Autodesk Inventor part; units mm, degrees
(part 2 of 2)
  spline S52 degree 2 poles (32.3634, 1.1115) (32.3453, 1.127) (32.3005, 1.138) (32.2753, 1.138) knots 0 0 0 1 2 2 2
  spline S53 degree 2 poles (32.2753, 1.138) (32.2539, 1.138) (32.2098, 1.127) (32.1903, 1.1192) knots 0 0 0 1 2 2 2
  spline S54 degree 2 poles (32.1903, 1.1192) (32.1903, 1.1141) (32.189, 1.0894) (32.189, 1.0706) knots 0 0 0 1 2 2 2
  spline S55 degree 2 poles (32.189, 1.0706) (32.189, 1.0013) (32.213, 0.9176) (32.2318, 0.8962) knots 0 0 0 1 2 2 2
  spline S56 degree 2 poles (32.2318, 0.8962) (32.2454, 0.8787) (32.2817, 0.8638) (32.3012, 0.8638) knots 0 0 0 1 2 2 2
  spline S57 degree 2 poles (32.3012, 0.8638) (32.3174, 0.8638) (32.355, 0.88) (32.368, 0.8962) knots 0 0 0 1 2 2 2
  line L247 (22.1174, -18.2657) -> (21.873, -18.2657)
  line L248 (21.873, -18.2657) -> (21.6506, -17.972)
  line L249 (21.6506, -17.972) -> (21.578, -17.972)
  line L250 (21.578, -17.972) -> (21.578, -18.2657)
  line L251 (21.578, -18.2657) -> (21.3784, -18.2657)
  line L252 (21.3784, -18.2657) -> (21.3784, -17.4657)
  line L253 (21.3784, -17.4657) -> (21.6999, -17.4657)
  spline S58 degree 2 poles (21.6999, -17.4657) (21.7667, -17.4657) (21.8652, -17.4826) (21.9074, -17.5085) knots 0 0 0 1 2 2 2
  spline S59 degree 2 poles (21.9074, -17.5085) (21.9502, -17.5357) (22.0007, -17.6206) (22.0007, -17.6855) knots 0 0 0 1 2 2 2
  spline S60 degree 2 poles (22.0007, -17.6855) (22.0007, -17.7769) (21.9177, -17.8916) (21.8484, -17.9253) knots 0 0 0 1 2 2 2
  line L254 (21.8484, -17.9253) -> (22.1174, -18.2657)
  spline S61 degree 2 poles (21.7946, -17.7108) (21.7946, -17.6803) (21.7712, -17.6368) (21.7446, -17.6252) knots 0 0 0 1 2 2 2
  spline S62 degree 2 poles (21.7446, -17.6252) (21.7258, -17.6174) (21.6798, -17.6129) (21.6455, -17.6129) knots 0 0 0 1 2 2 2
  line L255 (21.6455, -17.6129) -> (21.578, -17.6129)
  line L256 (21.578, -17.6129) -> (21.578, -17.8281)
  line L257 (21.578, -17.8281) -> (21.6357, -17.8281)
  spline S63 degree 2 poles (21.6357, -17.8281) (21.6772, -17.8281) (21.7362, -17.8177) (21.7563, -17.8015) knots 0 0 0 1 2 2 2
  spline S64 degree 2 poles (21.7563, -17.8015) (21.7758, -17.786) (21.7946, -17.7445) (21.7946, -17.7108) knots 0 0 0 1 2 2 2
  line L258 (22.7275, -18.2657) -> (22.1991, -18.2657)
  line L259 (22.1991, -18.2657) -> (22.1991, -18.1263)
  line L260 (22.1991, -18.1263) -> (22.3677, -18.1263)
  line L261 (22.3677, -18.1263) -> (22.3677, -17.703)
  line L262 (22.3677, -17.703) -> (22.1991, -17.703)
  line L263 (22.1991, -17.703) -> (22.1991, -17.5727)
  spline S65 degree 2 poles (22.1991, -17.5727) (22.2361, -17.5727) (22.3093, -17.5629) (22.3314, -17.5526) knots 0 0 0 1 2 2 2
  spline S66 degree 2 poles (22.3314, -17.5526) (22.3566, -17.5396) (22.3852, -17.4962) (22.3878, -17.4638) knots 0 0 0 1 2 2 2
  line L264 (22.3878, -17.4638) -> (22.5628, -17.4638)
  line L265 (22.5628, -17.4638) -> (22.5628, -18.1263)
  line L266 (22.5628, -18.1263) -> (22.7275, -18.1263)
  line L267 (22.7275, -18.1263) -> (22.7275, -18.2657)
  spline S67 degree 2 poles (22.1278, -9.1391) (22.1278, -9.1909) (22.0922, -9.283) (22.0565, -9.3154) knots 0 0 0 1 2 2 2
  spline S68 degree 2 poles (22.0565, -9.3154) (22.0163, -9.3517) (21.9068, -9.3861) (21.8354, -9.3861) knots 0 0 0 1 2 2 2
  spline S69 degree 2 poles (21.8354, -9.3861) (21.7823, -9.3861) (21.6889, -9.3783) (21.6533, -9.3705) knots 0 0 0 1 2 2 2
  line L268 (21.6533, -9.3705) -> (21.6533, -9.2084)
  line L269 (21.6533, -9.2084) -> (21.6714, -9.2084)
  spline S70 degree 2 poles (21.6714, -9.2084) (21.6954, -9.2182) (21.7479, -9.235) (21.7894, -9.235) knots 0 0 0 1 2 2 2
  spline S71 degree 2 poles (21.7894, -9.235) (21.8426, -9.235) (21.9003, -9.2052) (21.9119, -9.178) knots 0 0 0 1 2 2 2
  spline S72 degree 2 poles (21.9119, -9.178) (21.9243, -9.1514) (21.9268, -9.0827) (21.9268, -9.0399) knots 0 0 0 1 2 2 2
  line L270 (21.9268, -9.0399) -> (21.9268, -8.719)
  line L271 (21.9268, -8.719) -> (21.744, -8.719)
  line L272 (21.744, -8.719) -> (21.744, -8.5738)
  line L273 (21.744, -8.5738) -> (22.1278, -8.5738)
  line L274 (22.1278, -8.5738) -> (22.1278, -9.1391)
  line L275 (22.8695, -9.3738) -> (22.2815, -9.3738)
  line L276 (22.2815, -9.3738) -> (22.2815, -9.2435)
  spline S73 degree 2 poles (22.2815, -9.2435) (22.356, -9.1838) (22.4753, -9.0788) (22.52, -9.0315) knots 0 0 0 1 2 2 2
  spline S74 degree 2 poles (22.52, -9.0315) (22.579, -8.9699) (22.6315, -8.8759) (22.6315, -8.8266) knots 0 0 0 1 2 2 2
  spline S75 degree 2 poles (22.6315, -8.8266) (22.6315, -8.7708) (22.5648, -8.7112) (22.5051, -8.7112) knots 0 0 0 1 2 2 2
  spline S76 degree 2 poles (22.5051, -8.7112) (22.4747, -8.7112) (22.4202, -8.7261) (22.3923, -8.7378) knots 0 0 0 1 2 2 2
  spline S77 degree 2 poles (22.3923, -8.7378) (22.3651, -8.7501) (22.3262, -8.776) (22.3165, -8.7825) knots 0 0 0 1 2 2 2
  line L277 (22.3165, -8.7825) -> (22.3009, -8.7825)
  line L278 (22.3009, -8.7825) -> (22.3009, -8.6081)
  spline S78 degree 2 poles (22.3009, -8.6081) (22.3346, -8.5919) (22.4786, -8.5582) (22.5453, -8.5582) knots 0 0 0 1 2 2 2
  spline S79 degree 2 poles (22.5453, -8.5582) (22.688, -8.5582) (22.8345, -8.6853) (22.8345, -8.8) knots 0 0 0 1 2 2 2
  spline S80 degree 2 poles (22.8345, -8.8) (22.8345, -8.8707) (22.7677, -9.0068) (22.6905, -9.0846) knots 0 0 0 1 2 2 2
  spline S81 degree 2 poles (22.6905, -9.0846) (22.6419, -9.1326) (22.5505, -9.2072) (22.5304, -9.2227) knots 0 0 0 1 2 2 2
  line L279 (22.5304, -9.2227) -> (22.8695, -9.2227)
  line L280 (22.8695, -9.2227) -> (22.8695, -9.3738)
  spline S82 degree 2 poles (20.6809, -6.6196) (20.6809, -6.6715) (20.6452, -6.7636) (20.6096, -6.796) knots 0 0 0 1 2 2 2
  spline S83 degree 2 poles (20.6096, -6.796) (20.5694, -6.8323) (20.4598, -6.8667) (20.3885, -6.8667) knots 0 0 0 1 2 2 2
  spline S84 degree 2 poles (20.3885, -6.8667) (20.3353, -6.8667) (20.242, -6.8589) (20.2063, -6.8511) knots 0 0 0 1 2 2 2
  line L281 (20.2063, -6.8511) -> (20.2063, -6.689)
  line L282 (20.2063, -6.689) -> (20.2245, -6.689)
  spline S85 degree 2 poles (20.2245, -6.689) (20.2485, -6.6987) (20.301, -6.7156) (20.3425, -6.7156) knots 0 0 0 1 2 2 2
  spline S86 degree 2 poles (20.3425, -6.7156) (20.3956, -6.7156) (20.4533, -6.6858) (20.465, -6.6585) knots 0 0 0 1 2 2 2
  spline S87 degree 2 poles (20.465, -6.6585) (20.4773, -6.632) (20.4799, -6.5632) (20.4799, -6.5205) knots 0 0 0 1 2 2 2
  line L283 (20.4799, -6.5205) -> (20.4799, -6.1996)
  line L284 (20.4799, -6.1996) -> (20.2971, -6.1996)
  line L285 (20.2971, -6.1996) -> (20.2971, -6.0543)
  line L286 (20.2971, -6.0543) -> (20.6809, -6.0543)
  line L287 (20.6809, -6.0543) -> (20.6809, -6.6196)
  line L288 (21.3869, -6.8543) -> (20.8585, -6.8543)
  line L289 (20.8585, -6.8543) -> (20.8585, -6.7149)
  line L290 (20.8585, -6.7149) -> (21.0271, -6.7149)
  line L291 (21.0271, -6.7149) -> (21.0271, -6.2916)
  line L292 (21.0271, -6.2916) -> (20.8585, -6.2916)
  line L293 (20.8585, -6.2916) -> (20.8585, -6.1613)
  spline S88 degree 2 poles (20.8585, -6.1613) (20.8955, -6.1613) (20.9687, -6.1516) (20.9908, -6.1412) knots 0 0 0 1 2 2 2
  spline S89 degree 2 poles (20.9908, -6.1412) (21.016, -6.1282) (21.0446, -6.0848) (21.0472, -6.0524) knots 0 0 0 1 2 2 2
  line L294 (21.0472, -6.0524) -> (21.2222, -6.0524)
  line L295 (21.2222, -6.0524) -> (21.2222, -6.7149)
  line L296 (21.2222, -6.7149) -> (21.3869, -6.7149)
  line L297 (21.3869, -6.7149) -> (21.3869, -6.8543)
  line L298 (22.4777, 11.6258) -> (22.2333, 11.6258)
  line L299 (22.2333, 11.6258) -> (22.0109, 11.9195)
  line L300 (22.0109, 11.9195) -> (21.9383, 11.9195)
  line L301 (21.9383, 11.9195) -> (21.9383, 11.6258)
  line L302 (21.9383, 11.6258) -> (21.7386, 11.6258)
  line L303 (21.7386, 11.6258) -> (21.7386, 12.4258)
  line L304 (21.7386, 12.4258) -> (22.0602, 12.4258)
  spline S90 degree 2 poles (22.0602, 12.4258) (22.127, 12.4258) (22.2255, 12.4089) (22.2676, 12.383) knots 0 0 0 1 2 2 2
  spline S91 degree 2 poles (22.2676, 12.383) (22.3104, 12.3558) (22.361, 12.2709) (22.361, 12.206) knots 0 0 0 1 2 2 2
  spline S92 degree 2 poles (22.361, 12.206) (22.361, 12.1146) (22.278, 11.9999) (22.2086, 11.9662) knots 0 0 0 1 2 2 2
  line L305 (22.2086, 11.9662) -> (22.4777, 11.6258)
  spline S93 degree 2 poles (22.1548, 12.1807) (22.1548, 12.2112) (22.1315, 12.2547) (22.1049, 12.2663) knots 0 0 0 1 2 2 2
  spline S94 degree 2 poles (22.1049, 12.2663) (22.0861, 12.2741) (22.0401, 12.2786) (22.0057, 12.2786) knots 0 0 0 1 2 2 2
  line L306 (22.0057, 12.2786) -> (21.9383, 12.2786)
  line L307 (21.9383, 12.2786) -> (21.9383, 12.0634)
  line L308 (21.9383, 12.0634) -> (21.996, 12.0634)
  spline S95 degree 2 poles (21.996, 12.0634) (22.0375, 12.0634) (22.0965, 12.0738) (22.1166, 12.09) knots 0 0 0 1 2 2 2
  spline S96 degree 2 poles (22.1166, 12.09) (22.136, 12.1055) (22.1548, 12.147) (22.1548, 12.1807) knots 0 0 0 1 2 2 2
  line L309 (23.1234, 11.6258) -> (22.5354, 11.6258)
  line L310 (22.5354, 11.6258) -> (22.5354, 11.7561)
  spline S97 degree 2 poles (22.5354, 11.7561) (22.6099, 11.8158) (22.7292, 11.9208) (22.774, 11.9681) knots 0 0 0 1 2 2 2
  spline S98 degree 2 poles (22.774, 11.9681) (22.833, 12.0297) (22.8855, 12.1237) (22.8855, 12.173) knots 0 0 0 1 2 2 2
  spline S99 degree 2 poles (22.8855, 12.173) (22.8855, 12.2287) (22.8187, 12.2884) (22.759, 12.2884) knots 0 0 0 1 2 2 2
  spline S100 degree 2 poles (22.759, 12.2884) (22.7286, 12.2884) (22.6741, 12.2735) (22.6462, 12.2618) knots 0 0 0 1 2 2 2
  spline S101 degree 2 poles (22.6462, 12.2618) (22.619, 12.2495) (22.5801, 12.2235) (22.5704, 12.217) knots 0 0 0 1 2 2 2
  line L311 (22.5704, 12.217) -> (22.5548, 12.217)
  line L312 (22.5548, 12.217) -> (22.5548, 12.3914)
  spline S102 degree 2 poles (22.5548, 12.3914) (22.5885, 12.4076) (22.7325, 12.4414) (22.7992, 12.4414) knots 0 0 0 1 2 2 2
  spline S103 degree 2 poles (22.7992, 12.4414) (22.9419, 12.4414) (23.0884, 12.3143) (23.0884, 12.1995) knots 0 0 0 1 2 2 2
  spline S104 degree 2 poles (23.0884, 12.1995) (23.0884, 12.1289) (23.0216, 11.9927) (22.9445, 11.9149) knots 0 0 0 1 2 2 2
  spline S105 degree 2 poles (22.9445, 11.9149) (22.8958, 11.867) (22.8044, 11.7924) (22.7843, 11.7769) knots 0 0 0 1 2 2 2
  line L313 (22.7843, 11.7769) -> (23.1234, 11.7769)
  line L314 (23.1234, 11.7769) -> (23.1234, 11.6258)
  line L315 (40.1797, -0.8005) -> (40.45, -0.0005)
  line L316 (40.45, -0.0005) -> (40.6692, -0.0005)
  line L317 (40.6692, -0.0005) -> (40.9395, -0.8005)
  line L318 (40.9395, -0.8005) -> (40.7327, -0.8005)
  line L319 (40.7327, -0.8005) -> (40.6828, -0.6371)
  line L320 (40.6828, -0.6371) -> (40.4312, -0.6371)
  line L321 (40.4312, -0.6371) -> (40.3807, -0.8005)
  line L322 (40.3807, -0.8005) -> (40.1797, -0.8005)
  line L323 (40.6387, -0.4919) -> (40.557, -0.2274)
  line L324 (40.557, -0.2274) -> (40.4747, -0.4919)
  line L325 (40.4747, -0.4919) -> (40.6387, -0.4919)
  line L326 (41.0192, -0.8005) -> (41.0192, -0.0005)
  line L327 (41.0192, -0.0005) -> (41.5599, -0.0005)
  line L328 (41.5599, -0.0005) -> (41.5599, -0.1528)
  line L329 (41.5599, -0.1528) -> (41.2189, -0.1528)
  line L330 (41.2189, -0.1528) -> (41.2189, -0.2935)
  line L331 (41.2189, -0.2935) -> (41.5333, -0.2935)
  line L332 (41.5333, -0.2935) -> (41.5333, -0.4459)
  line L333 (41.5333, -0.4459) -> (41.2189, -0.4459)
  line L334 (41.2189, -0.4459) -> (41.2189, -0.6481)
  line L335 (41.2189, -0.6481) -> (41.5599, -0.6481)
  line L336 (41.5599, -0.6481) -> (41.5599, -0.8005)
  line L337 (41.5599, -0.8005) -> (41.0192, -0.8005)
  line L338 (42.2821, -0.8005) -> (41.6941, -0.8005)
  line L339 (41.6941, -0.8005) -> (41.6941, -0.6702)
  spline S106 degree 2 poles (41.6941, -0.6702) (41.7687, -0.6105) (41.888, -0.5055) (41.9327, -0.4582) knots 0 0 0 1 2 2 2
  spline S107 degree 2 poles (41.9327, -0.4582) (41.9917, -0.3966) (42.0442, -0.3026) (42.0442, -0.2533) knots 0 0 0 1 2 2 2
  spline S108 degree 2 poles (42.0442, -0.2533) (42.0442, -0.1976) (41.9774, -0.1379) (41.9178, -0.1379) knots 0 0 0 1 2 2 2
  spline S109 degree 2 poles (41.9178, -0.1379) (41.8873, -0.1379) (41.8329, -0.1528) (41.805, -0.1645) knots 0 0 0 1 2 2 2
  spline S110 degree 2 poles (41.805, -0.1645) (41.7778, -0.1768) (41.7389, -0.2027) (41.7291, -0.2092) knots 0 0 0 1 2 2 2
  line L340 (41.7291, -0.2092) -> (41.7136, -0.2092)
  line L341 (41.7136, -0.2092) -> (41.7136, -0.0348)
  spline S111 degree 2 poles (41.7136, -0.0348) (41.7473, -0.0186) (41.8912, 0.0151) (41.958, 0.0151) knots 0 0 0 1 2 2 2
  spline S112 degree 2 poles (41.958, 0.0151) (42.1006, 0.0151) (42.2471, -0.112) (42.2471, -0.2267) knots 0 0 0 1 2 2 2
  spline S113 degree 2 poles (42.2471, -0.2267) (42.2471, -0.2974) (42.1803, -0.4335) (42.1032, -0.5113) knots 0 0 0 1 2 2 2
  spline S114 degree 2 poles (42.1032, -0.5113) (42.0546, -0.5593) (41.9632, -0.6339) (41.9431, -0.6494) knots 0 0 0 1 2 2 2
  line L342 (41.9431, -0.6494) -> (42.2821, -0.6494)
  line L343 (42.2821, -0.6494) -> (42.2821, -0.8005)
  line L344 (44.752, -28.4247) -> (44.551, -28.4247)
  line L345 (44.551, -28.4247) -> (44.551, -28.07)
  line L346 (44.551, -28.07) -> (44.2781, -28.07)
  line L347 (44.2781, -28.07) -> (44.2781, -28.4247)
  line L348 (44.2781, -28.4247) -> (44.0771, -28.4247)
  line L349 (44.0771, -28.4247) -> (44.0771, -27.6247)
  line L350 (44.0771, -27.6247) -> (44.2781, -27.6247)
  line L351 (44.2781, -27.6247) -> (44.2781, -27.9177)
  line L352 (44.2781, -27.9177) -> (44.551, -27.9177)
  line L353 (44.551, -27.9177) -> (44.551, -27.6247)
  line L354 (44.551, -27.6247) -> (44.752, -27.6247)
  line L355 (44.752, -27.6247) -> (44.752, -28.4247)
  line L356 (45.4865, -27.7835) -> (45.1449, -28.4247)
  line L357 (45.1449, -28.4247) -> (44.9219, -28.4247)
  line L358 (44.9219, -28.4247) -> (45.2791, -27.7757)
  line L359 (45.2791, -27.7757) -> (44.8979, -27.7757)
  line L360 (44.8979, -27.7757) -> (44.8979, -27.6247)
  line L361 (44.8979, -27.6247) -> (45.4865, -27.6247)
  line L362 (45.4865, -27.6247) -> (45.4865, -27.7835)
  line L363 (44.8169, 27.8958) -> (44.6159, 27.8958)
  line L364 (44.6159, 27.8958) -> (44.6159, 28.2505)
  line L365 (44.6159, 28.2505) -> (44.3429, 28.2505)
  line L366 (44.3429, 28.2505) -> (44.3429, 27.8958)
  line L367 (44.3429, 27.8958) -> (44.142, 27.8958)
  line L368 (44.142, 27.8958) -> (44.142, 28.6958)
  line L369 (44.142, 28.6958) -> (44.3429, 28.6958)
  line L370 (44.3429, 28.6958) -> (44.3429, 28.4028)
  line L371 (44.3429, 28.4028) -> (44.6159, 28.4028)
  line L372 (44.6159, 28.4028) -> (44.6159, 28.6958)
  line L373 (44.6159, 28.6958) -> (44.8169, 28.6958)
  line L374 (44.8169, 28.6958) -> (44.8169, 27.8958)
  spline S115 degree 2 poles (45.5669, 28.1182) (45.5669, 28.067) (45.5241, 27.9782) (45.4833, 27.9458) knots 0 0 0 1 2 2 2
  spline S116 degree 2 poles (45.4833, 27.9458) (45.4425, 27.9133) (45.3251, 27.877) (45.2493, 27.877) knots 0 0 0 1 2 2 2
  spline S117 degree 2 poles (45.2493, 27.877) (45.1682, 27.877) (45.047, 27.914) (45.0081, 27.9458) knots 0 0 0 1 2 2 2
  spline S118 degree 2 poles (45.0081, 27.9458) (44.9699, 27.9775) (44.9335, 28.0637) (44.9335, 28.1117) knots 0 0 0 1 2 2 2
  spline S119 degree 2 poles (44.9335, 28.1117) (44.9335, 28.1804) (45.0094, 28.2719) (45.0814, 28.3023) knots 0 0 0 1 2 2 2
  line L375 (45.0814, 28.3023) -> (45.0814, 28.3056)
  spline S120 degree 2 poles (45.0814, 28.3056) (45.0107, 28.3399) (44.9549, 28.4378) (44.9549, 28.4981) knots 0 0 0 1 2 2 2
  spline S121 degree 2 poles (44.9549, 28.4981) (44.9549, 28.5422) (44.9938, 28.6193) (45.0321, 28.6498) knots 0 0 0 1 2 2 2
  spline S122 degree 2 poles (45.0321, 28.6498) (45.069, 28.679) (45.1812, 28.714) (45.2512, 28.714) knots 0 0 0 1 2 2 2
  spline S123 degree 2 poles (45.2512, 28.714) (45.3251, 28.714) (45.4353, 28.6822) (45.471, 28.6563) knots 0 0 0 1 2 2 2
  spline S124 degree 2 poles (45.471, 28.6563) (45.5073, 28.6304) (45.5462, 28.5552) (45.5462, 28.5117) knots 0 0 0 1 2 2 2
  spline S125 degree 2 poles (45.5462, 28.5117) (45.5462, 28.4547) (45.4801, 28.3633) (45.412, 28.3315) knots 0 0 0 1 2 2 2
  line L376 (45.412, 28.3315) -> (45.412, 28.3289)
  spline S126 degree 2 poles (45.412, 28.3289) (45.4917, 28.2965) (45.5669, 28.1915) (45.5669, 28.1182) knots 0 0 0 1 2 2 2
  spline S127 degree 2 poles (45.3686, 28.1098) (45.3686, 28.1493) (45.3348, 28.1908) (45.2804, 28.2174) knots 0 0 0 1 2 2 2
  spline S128 degree 2 poles (45.2804, 28.2174) (45.2648, 28.2245) (45.2058, 28.2472) (45.1831, 28.2569) knots 0 0 0 1 2 2 2
  spline S129 degree 2 poles (45.1831, 28.2569) (45.1624, 28.2362) (45.1293, 28.174) (45.1293, 28.137) knots 0 0 0 1 2 2 2
  spline S130 degree 2 poles (45.1293, 28.137) (45.1293, 28.0813) (45.2006, 28.0145) (45.2583, 28.0145) knots 0 0 0 1 2 2 2
  spline S131 degree 2 poles (45.2583, 28.0145) (45.2746, 28.0145) (45.3147, 28.0249) (45.3303, 28.0352) knots 0 0 0 1 2 2 2
  spline S132 degree 2 poles (45.3303, 28.0352) (45.3478, 28.0475) (45.3686, 28.0813) (45.3686, 28.1098) knots 0 0 0 1 2 2 2
  spline S133 degree 2 poles (45.3511, 28.4884) (45.3511, 28.5292) (45.2972, 28.5778) (45.2512, 28.5778) knots 0 0 0 1 2 2 2
  spline S134 degree 2 poles (45.2512, 28.5778) (45.2071, 28.5778) (45.1533, 28.5338) (45.1533, 28.5013) knots 0 0 0 1 2 2 2
  spline S135 degree 2 poles (45.1533, 28.5013) (45.1533, 28.4696) (45.1857, 28.43) (45.2201, 28.4138) knots 0 0 0 1 2 2 2
  spline S136 degree 2 poles (45.2201, 28.4138) (45.235, 28.406) (45.2765, 28.3898) (45.3109, 28.3769) knots 0 0 0 1 2 2 2
  spline S137 degree 2 poles (45.3109, 28.3769) (45.3316, 28.4041) (45.3511, 28.4553) (45.3511, 28.4884) knots 0 0 0 1 2 2 2
  line L377 (-8.7757, -9.36) -> (-8.5053, -8.56)
  line L378 (-8.5053, -8.56) -> (-8.2862, -8.56)
  line L379 (-8.2862, -8.56) -> (-8.0159, -9.36)
  line L380 (-8.0159, -9.36) -> (-8.2227, -9.36)
  line L381 (-8.2227, -9.36) -> (-8.2726, -9.1966)
  line L382 (-8.2726, -9.1966) -> (-8.5241, -9.1966)
  line L383 (-8.5241, -9.1966) -> (-8.5747, -9.36)
  line L384 (-8.5747, -9.36) -> (-8.7757, -9.36)
  line L385 (-8.3167, -9.0514) -> (-8.3983, -8.7869)
  line L386 (-8.3983, -8.7869) -> (-8.4807, -9.0514)
  line L387 (-8.4807, -9.0514) -> (-8.3167, -9.0514)
  line L388 (-7.9361, -9.36) -> (-7.9361, -8.56)
  line L389 (-7.9361, -8.56) -> (-7.3954, -8.56)
  line L390 (-7.3954, -8.56) -> (-7.3954, -8.7123)
  line L391 (-7.3954, -8.7123) -> (-7.7364, -8.7123)
  line L392 (-7.7364, -8.7123) -> (-7.7364, -8.853)
  line L393 (-7.7364, -8.853) -> (-7.422, -8.853)
  line L394 (-7.422, -8.853) -> (-7.422, -9.0053)
  line L395 (-7.422, -9.0053) -> (-7.7364, -9.0053)
  line L396 (-7.7364, -9.0053) -> (-7.7364, -9.2076)
  line L397 (-7.7364, -9.2076) -> (-7.3954, -9.2076)
  line L398 (-7.3954, -9.2076) -> (-7.3954, -9.36)
  line L399 (-7.3954, -9.36) -> (-7.9361, -9.36)
  line L400 (-6.7089, -9.36) -> (-7.2372, -9.36)
  line L401 (-7.2372, -9.36) -> (-7.2372, -9.2206)
  line L402 (-7.2372, -9.2206) -> (-7.0687, -9.2206)
  line L403 (-7.0687, -9.2206) -> (-7.0687, -8.7972)
  line L404 (-7.0687, -8.7972) -> (-7.2372, -8.7972)
  line L405 (-7.2372, -8.7972) -> (-7.2372, -8.6669)
  spline S138 degree 2 poles (-7.2372, -8.6669) (-7.2003, -8.6669) (-7.127, -8.6572) (-7.105, -8.6468) knots 0 0 0 1 2 2 2
  spline S139 degree 2 poles (-7.105, -8.6468) (-7.0797, -8.6339) (-7.0512, -8.5904) (-7.0486, -8.558) knots 0 0 0 1 2 2 2
  line L406 (-7.0486, -8.558) -> (-6.8735, -8.558)
  line L407 (-6.8735, -8.558) -> (-6.8735, -9.2206)
  line L408 (-6.8735, -9.2206) -> (-6.7089, -9.2206)
  line L409 (-6.7089, -9.2206) -> (-6.7089, -9.36)
  line L410 (-23.6301, 21.6881) -> (-23.831, 21.6881)
  line L411 (-23.831, 21.6881) -> (-23.831, 22.0427)
  line L412 (-23.831, 22.0427) -> (-24.104, 22.0427)
  line L413 (-24.104, 22.0427) -> (-24.104, 21.6881)
  line L414 (-24.104, 21.6881) -> (-24.3049, 21.6881)
  line L415 (-24.3049, 21.6881) -> (-24.3049, 22.4881)
  line L416 (-24.3049, 22.4881) -> (-24.104, 22.4881)
  line L417 (-24.104, 22.4881) -> (-24.104, 22.195)
  line L418 (-24.104, 22.195) -> (-23.831, 22.195)
  line L419 (-23.831, 22.195) -> (-23.831, 22.4881)
  line L420 (-23.831, 22.4881) -> (-23.6301, 22.4881)
  line L421 (-23.6301, 22.4881) -> (-23.6301, 21.6881)
  line L422 (-22.8683, 21.8748) -> (-22.9766, 21.8748)
  line L423 (-22.9766, 21.8748) -> (-22.9766, 21.6861)
  line L424 (-22.9766, 21.6861) -> (-23.1704, 21.6861)
  line L425 (-23.1704, 21.6861) -> (-23.1704, 21.8748)
  line L426 (-23.1704, 21.8748) -> (-23.5231, 21.8748)
  line L427 (-23.5231, 21.8748) -> (-23.5231, 22.0239)
  line L428 (-23.5231, 22.0239) -> (-23.1769, 22.4881)
  line L429 (-23.1769, 22.4881) -> (-22.9766, 22.4881)
  line L430 (-22.9766, 22.4881) -> (-22.9766, 22.0187)
  line L431 (-22.9766, 22.0187) -> (-22.8683, 22.0187)
  line L432 (-22.8683, 22.0187) -> (-22.8683, 21.8748)
  line L433 (-23.1704, 22.0187) -> (-23.1704, 22.291)
  line L434 (-23.1704, 22.291) -> (-23.3733, 22.0187)
  line L435 (-23.3733, 22.0187) -> (-23.1704, 22.0187)
  line L436 (-23.5442, -22.2943) -> (-23.7451, -22.2943)
  line L437 (-23.7451, -22.2943) -> (-23.7451, -21.9397)
  line L438 (-23.7451, -21.9397) -> (-24.0181, -21.9397)
  line L439 (-24.0181, -21.9397) -> (-24.0181, -22.2943)
  line L440 (-24.0181, -22.2943) -> (-24.219, -22.2943)
  line L441 (-24.219, -22.2943) -> (-24.219, -21.4943)
  line L442 (-24.219, -21.4943) -> (-24.0181, -21.4943)
  line L443 (-24.0181, -21.4943) -> (-24.0181, -21.7873)
  line L444 (-24.0181, -21.7873) -> (-23.7451, -21.7873)
  line L445 (-23.7451, -21.7873) -> (-23.7451, -21.4943)
  line L446 (-23.7451, -21.4943) -> (-23.5442, -21.4943)
  line L447 (-23.5442, -21.4943) -> (-23.5442, -22.2943)
  spline S140 degree 2 poles (-22.8122, -22.0518) (-22.8122, -22.1108) (-22.8557, -22.2074) (-22.8978, -22.2411) knots 0 0 0 1 2 2 2
  spline S141 degree 2 poles (-22.8978, -22.2411) (-22.94, -22.2749) (-23.0547, -22.3112) (-23.137, -22.3112) knots 0 0 0 1 2 2 2
  spline S142 degree 2 poles (-23.137, -22.3112) (-23.2304, -22.3112) (-23.3639, -22.28) (-23.4061, -22.2606) knots 0 0 0 1 2 2 2
  line L448 (-23.4061, -22.2606) -> (-23.4061, -22.0868)
  line L449 (-23.4061, -22.0868) -> (-23.3866, -22.0868)
  spline S143 degree 2 poles (-23.3866, -22.0868) (-23.3425, -22.1147) (-23.2239, -22.1562) (-23.1746, -22.1562) knots 0 0 0 1 2 2 2
  spline S144 degree 2 poles (-23.1746, -22.1562) (-23.1455, -22.1562) (-23.0774, -22.1458) (-23.0541, -22.129) knots 0 0 0 1 2 2 2
  spline S145 degree 2 poles (-23.0541, -22.129) (-23.0359, -22.1154) (-23.0139, -22.0758) (-23.0139, -22.0402) knots 0 0 0 1 2 2 2
  spline S146 degree 2 poles (-23.0139, -22.0402) (-23.0139, -22.0045) (-23.045, -21.9663) (-23.0709, -21.9572) knots 0 0 0 1 2 2 2
  spline S147 degree 2 poles (-23.0709, -21.9572) (-23.0968, -21.9481) (-23.1688, -21.9462) (-23.1967, -21.9462) knots 0 0 0 1 2 2 2
  line L450 (-23.1967, -21.9462) -> (-23.231, -21.9462)
  line L451 (-23.231, -21.9462) -> (-23.231, -21.8055)
  line L452 (-23.231, -21.8055) -> (-23.1993, -21.8055)
  spline S148 degree 2 poles (-23.1993, -21.8055) (-23.163, -21.8055) (-23.1014, -21.799) (-23.08, -21.7893) knots 0 0 0 1 2 2 2
  spline S149 degree 2 poles (-23.08, -21.7893) (-23.0586, -21.7789) (-23.0346, -21.7426) (-23.0346, -21.7115) knots 0 0 0 1 2 2 2
  spline S150 degree 2 poles (-23.0346, -21.7115) (-23.0346, -21.6868) (-23.0573, -21.6564) (-23.0735, -21.6479) knots 0 0 0 1 2 2 2
  spline S151 degree 2 poles (-23.0735, -21.6479) (-23.093, -21.6382) (-23.1448, -21.6317) (-23.163, -21.6317) knots 0 0 0 1 2 2 2
  spline S152 degree 2 poles (-23.163, -21.6317) (-23.1921, -21.6317) (-23.2537, -21.6454) (-23.2823, -21.6564) knots 0 0 0 1 2 2 2
  spline S153 degree 2 poles (-23.2823, -21.6564) (-23.3049, -21.6648) (-23.3542, -21.692) (-23.3659, -21.6992) knots 0 0 0 1 2 2 2
  line L453 (-23.3659, -21.6992) -> (-23.3827, -21.6992)
  line L454 (-23.3827, -21.6992) -> (-23.3827, -21.528)
  spline S154 degree 2 poles (-23.3827, -21.528) (-23.3413, -21.5105) (-23.2012, -21.4774) (-23.128, -21.4774) knots 0 0 0 1 2 2 2
  spline S155 degree 2 poles (-23.128, -21.4774) (-23.0566, -21.4774) (-22.9516, -21.5021) (-22.9147, -21.5261) knots 0 0 0 1 2 2 2
  spline S156 degree 2 poles (-22.9147, -21.5261) (-22.8738, -21.5514) (-22.833, -21.6291) (-22.833, -21.6778) knots 0 0 0 1 2 2 2
  spline S157 degree 2 poles (-22.833, -21.6778) (-22.833, -21.7465) (-22.9121, -21.8489) (-22.9769, -21.8638) knots 0 0 0 1 2 2 2
  line L455 (-22.9769, -21.8638) -> (-22.9769, -21.8716)
  spline S158 degree 2 poles (-22.9769, -21.8716) (-22.9484, -21.8755) (-22.8939, -21.8962) (-22.868, -21.9196) knots 0 0 0 1 2 2 2
  spline S159 degree 2 poles (-22.868, -21.9196) (-22.844, -21.9403) (-22.8122, -22.0065) (-22.8122, -22.0518) knots 0 0 0 1 2 2 2
  line L456 (-45.2027, -28.4422) -> (-45.4037, -28.4422)
  line L457 (-45.4037, -28.4422) -> (-45.4037, -28.0876)
  line L458 (-45.4037, -28.0876) -> (-45.6766, -28.0876)
  line L459 (-45.6766, -28.0876) -> (-45.6766, -28.4422)
  line L460 (-45.6766, -28.4422) -> (-45.8776, -28.4422)
  line L461 (-45.8776, -28.4422) -> (-45.8776, -27.6422)
  line L462 (-45.8776, -27.6422) -> (-45.6766, -27.6422)
  line L463 (-45.6766, -27.6422) -> (-45.6766, -27.9353)
  line L464 (-45.6766, -27.9353) -> (-45.4037, -27.9353)
  line L465 (-45.4037, -27.9353) -> (-45.4037, -27.6422)
  line L466 (-45.4037, -27.6422) -> (-45.2027, -27.6422)
  line L467 (-45.2027, -27.6422) -> (-45.2027, -28.4422)
  line L468 (-44.4863, -28.4422) -> (-45.0147, -28.4422)
  line L469 (-45.0147, -28.4422) -> (-45.0147, -28.3028)
  line L470 (-45.0147, -28.3028) -> (-44.8461, -28.3028)
  line L471 (-44.8461, -28.3028) -> (-44.8461, -27.8795)
  line L472 (-44.8461, -27.8795) -> (-45.0147, -27.8795)
  line L473 (-45.0147, -27.8795) -> (-45.0147, -27.7492)
  spline S160 degree 2 poles (-45.0147, -27.7492) (-44.9777, -27.7492) (-44.9045, -27.7395) (-44.8824, -27.7291) knots 0 0 0 1 2 2 2
  spline S161 degree 2 poles (-44.8824, -27.7291) (-44.8571, -27.7161) (-44.8286, -27.6727) (-44.826, -27.6403) knots 0 0 0 1 2 2 2
  line L474 (-44.826, -27.6403) -> (-44.651, -27.6403)
  line L475 (-44.651, -27.6403) -> (-44.651, -28.3028)
  line L476 (-44.651, -28.3028) -> (-44.4863, -28.3028)
  line L477 (-44.4863, -28.3028) -> (-44.4863, -28.4422)
  line L478 (-45.5229, 27.6078) -> (-45.7239, 27.6078)
  line L479 (-45.7239, 27.6078) -> (-45.7239, 27.9624)
  line L480 (-45.7239, 27.9624) -> (-45.9968, 27.9624)
  line L481 (-45.9968, 27.9624) -> (-45.9968, 27.6078)
  line L482 (-45.9968, 27.6078) -> (-46.1978, 27.6078)
  line L483 (-46.1978, 27.6078) -> (-46.1978, 28.4078)
  line L484 (-46.1978, 28.4078) -> (-45.9968, 28.4078)
  line L485 (-45.9968, 28.4078) -> (-45.9968, 28.1147)
  line L486 (-45.9968, 28.1147) -> (-45.7239, 28.1147)
  line L487 (-45.7239, 28.1147) -> (-45.7239, 28.4078)
  line L488 (-45.7239, 28.4078) -> (-45.5229, 28.4078)
  line L489 (-45.5229, 28.4078) -> (-45.5229, 27.6078)
  line L490 (-44.7709, 27.6078) -> (-45.3589, 27.6078)
  line L491 (-45.3589, 27.6078) -> (-45.3589, 27.7381)
  spline S162 degree 2 poles (-45.3589, 27.7381) (-45.2843, 27.7977) (-45.165, 27.9027) (-45.1203, 27.9501) knots 0 0 0 1 2 2 2
  spline S163 degree 2 poles (-45.1203, 27.9501) (-45.0613, 28.0117) (-45.0088, 28.1057) (-45.0088, 28.1549) knots 0 0 0 1 2 2 2
  spline S164 degree 2 poles (-45.0088, 28.1549) (-45.0088, 28.2107) (-45.0756, 28.2703) (-45.1352, 28.2703) knots 0 0 0 1 2 2 2
  spline S165 degree 2 poles (-45.1352, 28.2703) (-45.1657, 28.2703) (-45.2201, 28.2554) (-45.248, 28.2437) knots 0 0 0 1 2 2 2
  spline S166 degree 2 poles (-45.248, 28.2437) (-45.2752, 28.2314) (-45.3141, 28.2055) (-45.3239, 28.199) knots 0 0 0 1 2 2 2
  line L492 (-45.3239, 28.199) -> (-45.3394, 28.199)
  line L493 (-45.3394, 28.199) -> (-45.3394, 28.3734)
  spline S167 degree 2 poles (-45.3394, 28.3734) (-45.3057, 28.3896) (-45.1618, 28.4233) (-45.095, 28.4233) knots 0 0 0 1 2 2 2
  spline S168 degree 2 poles (-45.095, 28.4233) (-44.9524, 28.4233) (-44.8059, 28.2963) (-44.8059, 28.1815) knots 0 0 0 1 2 2 2
  spline S169 degree 2 poles (-44.8059, 28.1815) (-44.8059, 28.1108) (-44.8726, 27.9747) (-44.9498, 27.8969) knots 0 0 0 1 2 2 2
  spline S170 degree 2 poles (-44.9498, 27.8969) (-44.9984, 27.8489) (-45.0898, 27.7744) (-45.1099, 27.7588) knots 0 0 0 1 2 2 2
  line L494 (-45.1099, 27.7588) -> (-44.7709, 27.7588)
  line L495 (-44.7709, 27.7588) -> (-44.7709, 27.6078)
  point P0 (0, 0)
  point P1 (-35.75, 0)
  point P2 (-22.75, 13)
  point P3 (22.5, 15)
  point P4 (22.5, -15)
  point P5 (24, -9.75)
  dimension "d116" = 7
  dimension "d117" = 0.075
  dimension "d118" = 0.075
  dimension "d119" = 4.5
  dimension "d120" = 0.075
  dimension "d121" = 0.075
  dimension "d122" = 0.075
  dimension "d123" = 0.075
  dimension "d124" = 0.075
  dimension "d125" = 0.075
  dimension "d126" = 11
  dimension "d127" = 13
  dimension "d128" = 0.075
  dimension "d129" = 0.075
  dimension "d130" = 26
  dimension "d131" = 1.75
  dimension "d132" = 4.5
  dimension "d133" = 0.075
  dimension "d134" = 0.075
  dimension "d137" = 0.2
  dimension "d138" = 0.2
  dimension "d139" = 0.25
  dimension "d140" = 0.25
  dimension "d141" = 0.25
  dimension "d142" = 0.25
  dimension "d143" = 0.075
  dimension "d144" = 0.075
  dimension "d147" = 90
  dimension "d149" = 0.25
  dimension "d150" = 0.25
  dimension "d151" = 0.25
  dimension "d152" = 0.075
  dimension "d153" = 0.075
  constraints: 124 end point, 36 centre point, 26 parallel, 24 point on circle, 22 coincident, 15 equal radius, 12 perpendicular, 8 tangent, 5 midpoint, 4 point on line, 3 horizontal, 1 horizontal alignment, 1 vertical alignment, 77 other
  measures "d116" diameter of A72
  measures "d117" radial gap between concentric circles of A72 A73
  measures "d118" radial gap between concentric circles of A74 A72
  measures "d119" diameter of A98
  measures "d120" radial gap between concentric circles of A80 A98
  measures "d121" radial gap between concentric circles of A81 A98
  measures "d122" radial gap between concentric circles of A82 A99
  measures "d123" radial gap between concentric circles of A99 A83
  measures "d124" radial gap between concentric circles of A96 A100
  measures "d125" radial gap between concentric circles of A95 A100
  measures "d126" diameter of A100
  measures "d127" diameter of A99
  measures "d128" distance between parallel lines of L81 L85
  measures "d129" distance between parallel lines of L81 L89
  measures "d130" distance of L80.end L78.start
  measures "d131" horizontal distance of point (-22.75, 13) A30.centre
  measures "d132" distance between parallel lines of L91 L92
  measures "d133" radial gap between concentric circles of A102 A108
  measures "d134" radial gap between concentric circles of A110 A102
  measures "d137" distance between parallel lines of L105 L16
  measures "d138" distance between parallel lines of L18 L104
  measures "d139" distance between parallel lines of L75 L106
  measures "d140" distance between parallel lines of L108 L77
  measures "d141" distance between parallel lines of L37 L109
  measures "d142" distance between parallel lines of L107 L76
  measures "d143" distance between parallel lines of L109 L113
  measures "d144" distance between parallel lines of L109 L117
  measures "d149" distance between parallel lines of L18 L129
  measures "d150" distance between parallel lines of L128 L19
  measures "d151" distance between parallel lines of L21 L126
  measures "d152" distance between parallel lines of L129 L133
  measures "d153" distance between parallel lines of L137 L129
extrude "Extrusion5" add sketch "Sketch7" along normal blind 0.055 contours L8 L7 L132 L131 L101 L135 L136 L137 L0 A4 | A4 L0 L101 L133 L132 L7 L8 | L101 L104 L103 L0 | L0 L103 L133 L101 | L103 L137 A5 L0 | L0 A5 L137 L134 L1 L2 L130 L133 L103 | L133 L103 A39 L51 L101 | L51 A39 L103 A114 A112 L101 | L131 L103 L105 L101 | L101 A111 L100 A6 L102 A113 L103 L131 | L131 L130 L2 L1 A5 L134 L135 L103 | A114 L102 A6 L100 A112 A39 | L112 L113 L38 L117 L116 L41 | L41 L116 L115 L114 L43 L110 L111 L112 | L82 L85 L84 L83 A33 L87 L88 L89 L86 A39 | A39 L86 A29 L82 | A29 L86 L87 A31 L83 L82 | L113 L32 L117 L38 | L43 L114 L117 L32 L113 L110 | A31 L87 A33 L83 | L118 A14 L119 A15 | A15 L119 L122 L125 L121 L24 L120 L124 L123 L118 | L118 A27 L119 A14 | L118 L120 L24 L121 L119 A27 | L338 L339 S106 S107 S108 S109 S110 L340 L341 S111 S112 A23 S114 L342 L22 | L22 A23 L342 L343 L338 | S112 S113 S114 A23 | A64 | A65 | A74 | A76 | A82 | A85 | A88 | A92 | A94 | A96 | A108 L97 A107 L96 | S0 S1 S2 L198 L199 S3 S4 S5 L200 L201 L202 L203 L204 | S6 S7 S8 L205 L206 S9 S10 S11 S12 S13 L207 L208 L209 S14 S15 S16 S17 S18 S19 L210 L211 S20 S21 S22 S23 L212 S24 S25 | L213 L214 L215 L216 L217 L218 L219 L220 L221 L222 L223 L224 | S26 S27 S28 L225 L226 S29 S30 S31 S32 S33 S34 S35 L227 L228 L229 L230 L231 L232 S36 S37 S38 | L233 L234 L235 L236 L237 L238 L239 L240 L241 L242 L243 L244 | S39 S40 S41 S42 S43 S44 L245 L246 S45 S46 S47 S48 S49 | L247 L248 L249 L250 L251 L252 L253 S58 S59 S60 L254 | L258 L259 L260 L261 L262 L263 S65 S66 L264 L265 L266 L267 | S67 S68 S69 L268 L269 S70 S71 S72 L270 L271 L272 L273 L274 | L275 L276 S73 S74 S75 S76 S77 L277 L278 S78 S79 S80 S81 L279 L280 | S82 S83 S84 L281 L282 S85 S86 S87 L283 L284 L285 L286 L287 | L288 L289 L290 L291 L292 L293 S88 S89 L294 L295 L296 L297 | L298 L299 L300 L301 L302 L303 L304 S90 S91 S92 L305 | L309 L310 S97 S98 S99 S100 S101 L311 L312 S102 S103 S104 S105 L313 L314 | L315 L316 L317 L318 L319 L320 L321 L322 | L326 L327 L328 L329 L330 L331 L332 L333 L334 L335 L336 L337 | L344 L345 L346 L347 L348 L349 L350 L351 L352 L353 L354 L355 | L356 L357 L358 L359 L360 L361 L362 | L363 L364 L365 L366 L367 L368 L369 L370 L371 L372 L373 L374 | S115 S116 S117 S118 S119 L375 S120 S121 S122 S123 S124 S125 L376 S126 | L377 L378 L379 L380 L381 L382 L383 L384 | L388 L389 L390 L391 L392 L393 L394 L395 L396 L397 L398 L399 | L400 L401 L402 L403 L404 L405 S138 S139 L406 L407 L408 L409 | L410 L411 L412 L413 L414 L415 L416 L417 L418 L419 L420 L421 | L422 L423 L424 L425 L426 L427 L428 L429 L430 L431 L432 | L436 L437 L438 L439 L440 L441 L442 L443 L444 L445 L446 L447 | S140 S141 S142 L448 L449 S143 S144 S145 S146 S147 L450 L451 L452 S148 S149 S150 S151 S152 S153 L453 L454 S154 S155 S156 S157 L455 S158 S159 | L456 L457 L458 L459 L460 L461 L462 L463 L464 L465 L466 L467 | L468 L469 L470 L471 L472 L473 S160 S161 L474 L475 L476 L477 | L478 L479 L480 L481 L482 L483 L484 L485 L486 L487 L488 L489 | L490 L491 S162 S163 S164 S165 S166 L492 L493 S167 S168 S169 S170 L494 L495
ref_plane "Work Plane1" through (0.985, 0, 0) normal (1, 0, 0) x (0, 0, -1)
sketch "Sketch8" plane through (0.985, 0, 0) normal (1, 0, 0) x (0, 0, -1)
  line L0 (20.9948, -4.773) -> (19.227, -3.0052) projected
  line L1 (19.227, -3.0052) -> (16.7522, -5.4801) projected
  line L2 (16.7522, -5.4801) -> (18.5199, -7.2478) projected
  line L3 (18.5199, -7.2478) -> (20.9948, -4.773) projected
  line L4 (31.2478, -5.4801) -> (28.773, -3.0052) projected
  line L5 (28.773, -3.0052) -> (27.0052, -4.773) projected
  line L6 (27.0052, -4.773) -> (27.8347, -5.6024) projected
  line L7 (27.8347, -5.6024) -> (29.4801, -7.2478) projected
  line L8 (29.4801, -7.2478) -> (30.0347, -6.6933) projected
  line L9 (30.0347, -6.6933) -> (31.2478, -5.4801) projected
  line L10 (24.25, -13) -> (27.25, -13) projected
  line L11 (27.25, -13) -> (27.25, -10) projected
  line L12 (27.25, -10) -> (24.25, -10) projected
  line L13 (24.25, -10) -> (24.25, -13) projected
  line L14 (20.75, -13) -> (23.75, -13) projected
  line L15 (23.75, -13) -> (23.75, -10) projected
  line L16 (23.75, -10) -> (20.75, -10) projected
  line L17 (20.75, -10) -> (20.75, -13) projected
  line L18 (20.9948, -4.773) -> (19.227, -3.0052) projected
  point P0 (0, 0)
  point P1 (20.1109, -3.8891)
  point P2 (22.25, -10)
  point P3 (25.75, -10)
  point P4 (27.8891, -3.8891)
  constraints: 4 midpoint
ref_plane "Work Plane2" through (-2.95, 0, 0) normal (-1, 0, 0) x (0, 0, 1)
sketch "Sketch9" plane through (-2.95, 0, 0) normal (-1, 0, 0) x (0, 0, 1)
  line L0 (-10, 14.6) -> (-11, 14.6)
  line L1 (-10, 13.2) -> (-11, 13.2)
  point P0 (0, 0)
  dimension "d156" = 1
  dimension "d157" = 1.4
  dimension "d158" = 10
  dimension "d159" = 13.2
  constraints: 4 end point, 2 horizontal, 2 vertical alignment
  measures "d156" distance of L0.start L0.end
  measures "d157" distance between parallel lines of L1 L0
  measures "d158" horizontal distance of L0.start point (0, 0)
  measures "d159" distance from line of L1 point (0, 0)
body "Solid1"
